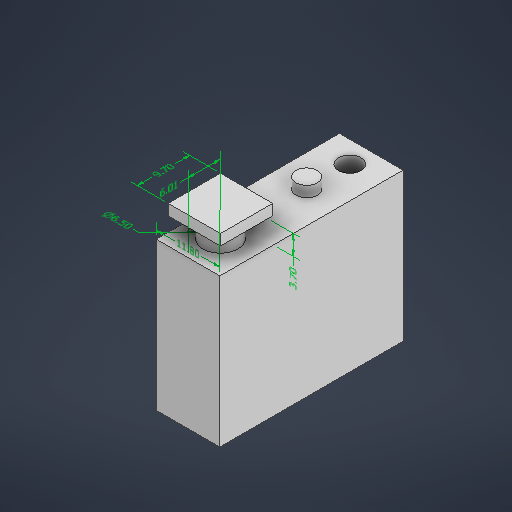
# Autodesk Inventor part: MS-1.5A Servo
Saved by Autodesk Inventor 2026.1 (Build 301233020, 233B)
## iProperties
Created: 2025-10-30
Part Number: MS-1.5A Servo
Material: Generic
Document SubType Name: Modeling
Designer: Asus
Density: 1 g/cm^3
Appearance: Default
Author: Asus
Autodesk Inventor part; units mm, degrees
ref_plane "YZ Plane" through (0, 0, 0) normal (1, 0, 0) x (0, 1, 0)
ref_plane "XZ Plane" through (0, 0, 0) normal (0, 1, 0) x (-1, 0, 0)
ref_plane "XY Plane" through (0, 0, 0) normal (0, 0, 1) x (1, 0, 0)
sketch "Sketch1" plane through (0, 0, 0) normal (0, 1, 0) x (-1, 0, 0)
  line L0 (0, 0) -> (11.8, 0)
  line L1 (11.8, 0) -> (11.8, -34)
  line L2 (11.8, -34) -> (0, -34)
  line L3 (0, -34) -> (0, 0)
  circle A0 centre (5.9, -30.01) radius 2.075
  dimension "d0" = 11.8
  dimension "d1" = 34
  dimension "d2" = 4.15
  dimension "d3" = 30.01
  constraints: 8 end point, 2 parallel, 1 centre point, 1 horizontal, 1 perpendicular
  measures "d0" distance of L1.end L2.end
  measures "d1" distance of L0.end L1.end
  measures "d2" diameter of A0
  measures "d3" distance from line of L0 A0.centre
extrude "Extrusion1" add sketch "Sketch1" along normal blind 27.5
sketch "Sketch2" plane through (0, 27.5, 0) normal (0, 1, 0) x (1, 0, 0)
  circle A0 centre (-5.9, 6.01) radius 3.25
  line L0 (-11.8, 0) -> (0, 0) projected
  line L1 (0, 0) -> (0, 34) projected
  dimension "d6" = 6.5
  dimension "d7" = 6.01
  dimension "d8" = 5.9
  constraints: 1 centre point
  measures "d6" diameter of A0
  measures "d7" distance from line of A0.centre L0
  measures "d8" distance from line of L1 A0.centre
extrude "Extrusion2" add sketch "Sketch2" along normal blind 5.7
sketch "Sketch3" plane through (-5.9, 33.2, -6.01) normal (0, 1, 0) x (1, 0, 0)
  line L0 (-4.85, -4.85) -> (4.85, -4.85)
  line L1 (4.85, -4.85) -> (4.85, 4.85)
  line L2 (4.85, 4.85) -> (-4.85, 4.85)
  line L3 (-4.85, 4.85) -> (-4.85, -4.85)
  line L4 (-4.85, -4.85) -> (4.85, 4.85) construction
  line L5 (4.85, -4.85) -> (-4.85, 4.85) construction
  point P0 (5.9, -6.01)
  point P1 (0, 0)
  dimension "d11" = 9.7
  dimension "d12" = 9.7
  constraints: 12 end point, 2 midpoint, 2 parallel, 1 horizontal, 1 perpendicular
  measures "d11" distance of L2.end L1.end
  measures "d12" distance of L1.end L0.end
extrude "Extrusion3" add sketch "Sketch3" against normal blind 2
sketch "Sketch4" plane through (0, 0, 0) normal (0, -1, 0) x (1, 0, 0)
  circle A0 centre (-5.9, -6.01) radius 3.25 projected
  circle A1 centre (-5.9, -6.01) radius 1.975
  point P0 (0, 0)
  dimension "d24" = 3.95
  constraints: 1 centre point, 1 coincident
  measures "d24" diameter of A1
extrude "Extrusion4" add sketch "Sketch4" along normal blind 2 contours A1
sketch "Sketch5" plane through (0, 27.5, 0) normal (0, 1, 0) x (1, 0, 0)
  circle A0 centre (-5.9, 22.01) radius 1.975
  circle A1 centre (-5.9, 30.01) radius 2.075 projected
  point P0 (0, 0)
  dimension "d27" = 3.95
  dimension "d28" = 8
  constraints: 1 centre point
  measures "d27" diameter of A0
  measures "d28" distance of A0.centre A1.centre
extrude "Extrusion5" add sketch "Sketch5" along normal blind 2 contours A0
sketch "Sketch6" plane through (0, 0, 0) normal (0, -1, 0) x (1, 0, 0)
  circle A0 centre (-5.9, -22.01) radius 1.975 projected
  circle A1 centre (-5.9, -22.01) radius 1.975
  point P0 (0, 0)
  constraints: 1 centre point, 1 coincident
extrude "Extrusion6" add sketch "Sketch6" along normal blind 2
body "Solid1"
